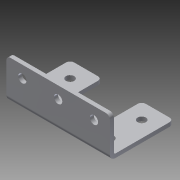
# Autodesk Inventor part: Chassis Bumper Mount - front - end - large
Saved by Autodesk Inventor 2013 (Build 170138000, 138)
## iProperties
Created: 2013-01-25
Part Number: Chassis Bumper Mount - front - end - large
Material: Aluminum 6061
Document SubType Name: Sheet Metal
Designer: Moses
Mass: 45.8415 g
Surface Area: 123.955 cm^2
Volume: 16.9157 cm^3
Density: 2.71 g/cm^3
Sheet Metal Rule: Default
Author: Moses
Autodesk Inventor part; units mm, degrees
ref_plane "YZ Plane" through (0, 0, 0) normal (1, 0, 0) x (0, 1, 0)
ref_plane "XZ Plane" through (0, 0, 0) normal (0, 1, 0) x (-1, 0, 0)
ref_plane "XY Plane" through (0, 0, 0) normal (0, 0, 1) x (1, 0, 0)
sketch "Sketch1" plane through (0, 0, 0) normal (0, 1, 0) x (-1, 0, 0)
  line L0 (0, 0) -> (82.55, 0)
  line L1 (82.55, 0) -> (82.55, 50.8)
  line L2 (82.55, 50.8) -> (0, 50.8)
  line L3 (0, 50.8) -> (0, 0)
  line L4 (12.7, 50.8) -> (12.7, 0) construction
  line L5 (69.85, 0) -> (69.85, 50.8) construction
  circle A0 centre (12.7, 12.7) radius 3.302
  circle A1 centre (69.85, 12.7) radius 3.302
  circle A2 centre (12.7, 38.1) radius 3.302
  circle A3 centre (69.85, 38.1) radius 3.302
  circle A4 centre (31.75, 38.1) radius 3.302
  circle A5 centre (50.8, 38.1) radius 3.302
  line L6 (12.7, 38.1) -> (69.85, 38.1) construction
  line L7 (25.4, 0) -> (25.4, 25.4)
  line L8 (25.4, 25.4) -> (57.15, 25.4)
  line L9 (57.15, 25.4) -> (57.15, 0)
  line L10 (41.275, 25.4) -> (41.275, 0) construction
  dimension "d0" = 82.55
  dimension "d2" = 12.7
  dimension "d3" = 12.7
  dimension "d4" = 6.604
  dimension "d5" = 19.05
  dimension "d6" = 19.05
  dimension "d7" = 12.7
  dimension "d8" = 25.4
  dimension "d9" = 25.4
  dimension "d10" = 12.7
  dimension "d11" = 12.7
  dimension "d12" = 25.4
  measures "d0" distance of L0.start L0.end
  measures "d2" distance between parallel lines of L4 L3
  measures "d3" distance between parallel lines of L1 L5
  measures "d4" diameter of A2
  measures "d5" distance of A4.centre L6.start
  measures "d6" distance of L6.end A5.centre
  measures "d7" distance from line of L2 L6.start
  measures "d8" distance of L6.start A0.centre
  measures "d9" distance of A1.centre L6.end
  measures "d10" distance from line of L0 A0.centre
  measures "d11" distance between parallel lines of L5 L9
  measures "d12" distance between parallel lines of L0 L8
extrude "Plate1" add sketch "Sketch1" along normal blind 3.175 contours L3 L2 L1 L0 L9 L8 L7
sketch "Sketch2" plane through (0, 0, 47.625) normal (0, 0, 1) x (1, 0, 0)
  line L0 (-82.55, 0) -> (0, 0)
  line L1 (0, 0) -> (0, 31.75)
  line L2 (0, 31.75) -> (-82.55, 31.75)
  line L3 (-82.55, 31.75) -> (-82.55, 0)
  constraints: 6 end point, 1 horizontal, 1 perpendicular, 1 vertical
edge flange "Flange1" height 31.75 angle 90 thickness 3.175 bend radius 1.27 thickness toward (0, 0, 1) relief straight relief width 3.175 relief depth 1.5875 edges at (-41.275, 3.175, 50.8) wall of the first edge with corners at (-82.55, 0, 47.625) (0, 0, 47.625) (0, 31.75, 47.625) (-82.55, 31.75, 47.625)
bend "Bend1"
corner "Corner1"
sketch "Sketch3" plane through (-82.55, 31.75, 50.8) normal (0, 0, 1) x (1, 0, 0)
  line L0 (82.55, 0) -> (82.55, -27.305) projected
  line L1 (0, 0) -> (82.55, 0) projected
  line L2 (0, -27.305) -> (0, 0) projected
  circle A0 centre (12.7, -9.525) radius 3.302
  circle A1 centre (41.275, -9.525) radius 3.302
  circle A2 centre (69.85, -9.525) radius 3.302
  line L3 (12.7, -9.525) -> (69.85, -9.525) construction
  line L4 (82.55, -31.75) -> (0, -31.75) construction
  line L5 (41.275, 0) -> (41.275, -31.75) construction
  dimension "d24" = 6.604
  dimension "d26" = 12.7
  dimension "d27" = 22.225
  constraints: 4 end point, 3 centre point, 3 midpoint, 2 equal radius, 1 coincident, 1 perpendicular, 1 point on line
  measures "d24" diameter of A0
  measures "d26" distance from line of L0 L3.end
  measures "d27" distance between parallel lines of L4 L3
extrude "Cut1" cut sketch "Sketch3" against normal blind 3.175
fillet "Corner Round1" radius 3.175 8 edges at (-82.55, 31.75, 49.2125) (0, 31.75, 49.2125) (-25.4, 1.5875, 0) (0, 1.5875, 0) (-57.15, 1.5875, 0) (-82.55, 1.5875, 0) (-57.15, 1.5875, 25.4) (-25.4, 1.5875, 25.4)
equation "\"d11\" = d2"
equation "\"d28\" = Thickness"
equation "\"d14\" = BendReliefWidth"
equation "\"d15\" = BendReliefDepth"
equation "\"d16\" = MinimumRemnant"
equation "\"d17\" = BendRadius"
equation "\"d21\" = CornerReliefSize"
equation "\"d22\" = GapSize"
equation "\"d23\" = JacobiRadiusSize"
equation "\"BendRadius\" = Thickness"
equation "\"BendReliefWidth\" = Thickness"
equation "\"BendReliefDepth\" = 0.5 * Thickness"
equation "\"CornerReliefSize\" = 4 * Thickness"
equation "\"MinimumRemnant\" = 2 * Thickness"
equation "\"TransitionRadius\" = BendRadius"
equation "\"JacobiRadiusSize\" = BendRadius"
equation "\"GapSize\" = Thickness"
equation "\"d13\" = BendRadius"
equation "\"Thickness\" = 3.175"
body "Solid1"
